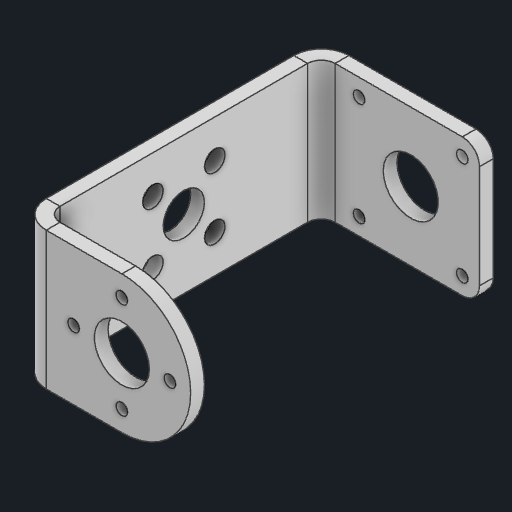
# Autodesk Inventor part: Part3
Saved by Autodesk Inventor 2025.2 (Build 292293000, 293)
## iProperties
Created: 2025-07-26
Part Number: Part3
Material: Generic
Document SubType Name: Sheet Metal
Designer: valer
Density: 1 g/cm^3
Sheet Metal Rule: Default
Appearance: Default
Author: valer
Autodesk Inventor part; units mm, degrees
ref_plane "YZ Plane" through (0, 0, 0) normal (1, 0, 0) x (0, 1, 0)
ref_plane "XZ Plane" through (0, 0, 0) normal (0, 1, 0) x (-1, 0, 0)
ref_plane "XY Plane" through (0, 0, 0) normal (0, 0, 1) x (1, 0, 0)
sketch "Sketch1" plane through (0, 0, 0) normal (0, 0, 1) x (1, 0, 0)
  line L0 (2.5, 10) -> (37.5, 10) construction
  line L1 (0, -7.5) -> (0, 7.5) construction
  line L2 (37.5, -10) -> (2.5, -10) construction
  circle A0 centre (10, -7) radius 0.85
  circle A1 centre (10, 7) radius 0.85
  circle A2 centre (3, 0) radius 0.85
  circle A3 centre (10, 0) radius 10
  line L3 (10, 7) -> (10, -7) construction
  circle A4 centre (17, 0) radius 0.85
  line L4 (10, 10) -> (-5, 10)
  line L5 (-5, 10) -> (-5, -10)
  line L6 (-5, -10) -> (10, -10)
  line L7 (10, -10) -> (10, 10)
  line L8 (10, 0) -> (20, 0)
  point P0 (0, 0)
  dimension "d0" = 25
  measures "d0" distance from line of L5 L8.end
extrude "Plate1" add sketch "Sketch1" along normal blind 2 contours A0 L7 L8 A4 A3 | A0 L7 A3 A1 | L7 A1 A3 L8 A4 | L6 L5 L4 A3
sketch "Sketch2" plane through (-3, 10, 2) normal (-1, 0, 0) x (0, -1, 0)
  line L0 (20, 0) -> (0, 0)
  line L1 (0, 0) -> (0, -44)
  line L2 (0, -44) -> (20, -44)
  line L3 (20, -44) -> (20, 0)
  constraints: 6 end point, 1 horizontal, 1 perpendicular, 1 vertical
edge flange "Flange1" height 44 angle 90 thickness 2 bend radius 2 thickness toward (-1, 0, 0) relief tear relief width 2 relief depth 1 edges at (-5, 0, 0) wall of the first edge with corners at (-3, -10, 2) (-3, 10, 2) (-3, 10, -42) (-3, -10, -42)
bend "Bend1"
corner "Corner1"
sketch "Sketch3" plane through (-5, 10, -40) normal (0, 0, -1) x (-1, 0, 0)
  line L0 (0, -20) -> (0, 0)
  line L1 (0, 0) -> (-25, 0)
  line L2 (-25, 0) -> (-25, -20)
  line L3 (-25, -20) -> (0, -20)
  constraints: 6 end point, 1 horizontal, 1 perpendicular, 1 vertical
edge flange "Flange2" height 25 angle 90 thickness 2 bend radius 2 thickness toward (0, 0, -1) relief tear relief width 2 relief depth 1 edges at (-3, 0, -42) wall of the first edge with corners at (-5, -10, -40) (-5, 10, -40) (20, 10, -40) (20, -10, -40)
bend "Bend2"
corner "Corner2"
fillet "Fillet1" radius 2.5 2 edges at (20, 10, -41) (20, -10, -41)
sketch "Sketch4" plane through (-1, -10, -42) normal (0, 0, -1) x (-1, 0, 0)
  circle A0 centre (-18.5, 2.5) radius 0.85 projected
  circle A1 centre (-18.5, 17.5) radius 0.85 projected
  circle A2 centre (-3.5, 17.5) radius 0.85 projected
  circle A3 centre (-3.5, 2.5) radius 0.85 projected
  point P0 (-1, 10)
extrude "Cut1" cut sketch "Sketch4" against normal blind 2
sketch "Sketch5" plane through (-5, -10, -2) normal (-1, 0, 0) x (0, 0, 1)
  line L0 (-36, 20) -> (0, 20) construction
  line L1 (-18, 20) -> (-18, 0) construction
  line L2 (0, 0) -> (-36, 0) construction
  circle A0 centre (-18, 10) radius 3
  line L3 (-22.5, 14.5) -> (-13.5, 14.5) construction
  line L4 (-13.5, 14.5) -> (-13.5, 5.5) construction
  line L5 (-13.5, 5.5) -> (-22.5, 5.5) construction
  line L6 (-22.5, 5.5) -> (-22.5, 14.5) construction
  line L7 (-22.5, 14.5) -> (-13.5, 5.5) construction
  circle A1 centre (-13.5, 14.5) radius 1.5
  circle A2 centre (-22.5, 14.5) radius 1.5
  circle A3 centre (-22.5, 5.5) radius 1.5
  circle A4 centre (-13.5, 5.5) radius 1.5
  point P0 (2, 10)
  dimension "d25" = 6
  dimension "d26" = 9
  dimension "d27" = 3
  constraints: 12 end point, 5 centre point, 4 coincident, 4 midpoint, 3 equal radius, 2 parallel, 2 perpendicular, 1 horizontal
  measures "d25" diameter of A0
  measures "d26" distance of L3.start L3.end
  measures "d27" diameter of A1
extrude "Cut2" cut sketch "Sketch5" against normal blind 2
sketch "Sketch6" plane through (0, 0, 2) normal (0, 0, 1) x (1, 0, 0)
  arc A0 (10, -10) -> (10, 10) centre (10, 0) ccw construction
  circle A1 centre (10, 0) radius 4
  point P0 (0, 0)
  dimension "d30" = 8
  constraints: 1 centre point, 1 coincident
  measures "d30" diameter of A1
extrude "Cut3" cut sketch "Sketch6" against normal through all
equation "\"d23\" = Thickness"
equation "\"d28\" = Thickness"
equation "\"d31\" = Thickness"
equation "\"d1\" = Thickness"
equation "\"d2\" = BendReliefWidth"
equation "\"d3\" = BendReliefDepth"
equation "\"d4\" = MinimumRemnant"
equation "\"d5\" = TransitionRadius"
equation "\"d8\" = BendRadius"
equation "\"d9\" = CornerReliefSize"
equation "\"d10\" = GapSize"
equation "\"d11\" = JacobiRadiusSize"
equation "\"d12\" = BendReliefWidth"
equation "\"d13\" = BendReliefDepth"
equation "\"d14\" = MinimumRemnant"
equation "\"d15\" = TransitionRadius"
equation "\"d18\" = BendRadius"
equation "\"d19\" = CornerReliefSize"
equation "\"d20\" = GapSize"
equation "\"d21\" = JacobiRadiusSize"
equation "\"BendRadius\" = Thickness"
equation "\"BendReliefWidth\" = Thickness"
equation "\"BendReliefDepth\" = 0.5 * Thickness"
equation "\"CornerReliefSize\" = 4 * Thickness"
equation "\"MinimumRemnant\" = 2 * Thickness"
equation "\"TransitionRadius\" = BendRadius"
equation "\"JacobiRadiusSize\" = BendRadius"
equation "\"GapSize\" = Thickness"
equation "\"Thickness\" = 2"
body "Solid1"
